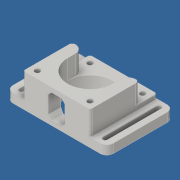
# Autodesk Inventor part: rotNema23Mount
Saved by Autodesk Inventor 2016 (Build 200138000, 138)
## iProperties
Created: 2015-10-04
Part Number: rotNema23Mount
Material: ABS-Kunststoff
Document SubType Name: Modeling
Designer: 4ndreas
Density: 1.06 g/cm^3
Appearance: Glatt - weiß
Mass: 62.6709 g
Surface Area: 197.225 cm^2
Volume: 59.1235 cm^3
Author: 4ndreas
Autodesk Inventor part; units mm, degrees
ref_plane "YZ Plane" through (0, 0, 0) normal (1, 0, 0) x (0, 1, 0)
sketch "Skizze1" plane through (0, 0, 0) normal (0, 0, 1) x (1, 0, 0)
  line L0 (-45, -30) -> (45, -30)
  line L1 (45, -30) -> (45, 30)
  line L2 (45, 30) -> (-45, 30)
  line L3 (-45, 30) -> (-45, -30)
  line L4 (-45, -30) -> (45, 30) construction
  line L5 (45, -30) -> (-45, 30) construction
  point P0 (0, 0)
  dimension "d0" = 60
  dimension "d1" = 90
  constraints: 12 end point, 2 midpoint, 2 parallel, 1 horizontal, 1 perpendicular
  measures "d0" distance between parallel lines of L0 L2
  measures "d1" distance between parallel lines of L3 L1
extrude "Extrusion1" add sketch "Skizze1" along normal blind 6
sketch "Skizze2" plane through (0, 0, 6) normal (0, 0, 1) x (1, 0, 0)
  line L0 (-30, -30) -> (30, -30)
  line L1 (30, -30) -> (30, 30)
  line L2 (30, 30) -> (-30, 30)
  line L3 (-30, 30) -> (-30, -30)
  line L4 (-30, -30) -> (30, 30) construction
  line L5 (30, -30) -> (-30, 30) construction
  line L6 (-45, -30) -> (45, -30) projected
  line L7 (45, -30) -> (45, 30) projected
  line L8 (45, 30) -> (-45, 30) projected
  line L9 (-45, 30) -> (-45, -30) projected
  line L10 (45, 30) -> (-45, 30) projected
  point P0 (0, 0)
  constraints: 12 end point, 2 midpoint, 2 parallel, 2 perpendicular, 1 collinear, 1 horizontal
sketch "Skizze3" plane through (0, 0, 0) normal (0, 0, -1) x (-1, 0, 0)
  line L0 (23.57, 23.57) -> (-23.57, 23.57) construction
  line L1 (-23.57, 23.57) -> (-23.57, -23.57) construction
  line L2 (-23.57, -23.57) -> (23.57, -23.57) construction
  line L3 (23.57, -23.57) -> (23.57, 23.57) construction
  line L4 (23.57, 23.57) -> (-23.57, -23.57) construction
  line L5 (-23.57, 23.57) -> (23.57, -23.57) construction
  point P0 (0, 0)
  dimension "d4" = 47.14
  constraints: 12 end point, 2 midpoint, 2 parallel, 2 perpendicular, 1 horizontal
  measures "d4" distance between parallel lines of L0 L2
extrude "Extrusion2" add sketch "Skizze2" along normal blind 14 contours L3 L2 L1 L0
hole "Bohrung1" at (-23.57, -23.57, 0) at (23.57, -23.57, 0) at (23.57, 23.57, 0) at (-23.57, 23.57, 0) direction (0, 0, 1) diameter 4.2 end through all
sketch "Skizze5" plane through (0, 0, 20) normal (0, 0, 1) x (1, 0, 0)
  circle A0 centre (0, 0) radius 20
  line L0 (-30, -30) -> (30, -30) projected
  line L1 (30, -30) -> (30, 30) projected
  line L2 (30, 30) -> (-30, 30) projected
  line L3 (-30, 30) -> (-30, -30) projected
  circle A1 centre (23.57, 23.57) radius 10
  circle A2 centre (-23.57, 23.57) radius 10
  line L4 (20, 0) -> (20, 14.229)
  line L5 (-20, 0) -> (-20, 14.229)
  line L6 (15.9113, 30) -> (-15.9113, 30)
  circle A3 centre (23.57, 23.57) radius 2.1 projected
  circle A4 centre (-23.57, 23.57) radius 2.1 projected
  dimension "d17" = 40
  dimension "d18" = 20
  constraints: 6 end point, 6 point on circle, 5 coincident, 3 centre point, 2 point on line, 2 tangent, 1 equal radius, 1 parallel, 1 vertical
  measures "d17" diameter of A0
  measures "d18" diameter of A1
extrude "Extrusion4" cut sketch "Skizze5" against normal blind 8 contours A0 | A0 L5 A2 L2 A1 L4 | A1 L2 L1 | A2 L3 L2 | A1 L1 L2 | A2 L2 L3 | A3 | A4
fillet "Rundung1" radius 7 2 edges at (20, 14.229, 16) (-20, 14.229, 16)
fillet "Rundung1" radius 3 2 edges at (-30, 15.9113, 16) (30, 15.9113, 16)
sketch "Skizze6" plane through (0, 0, 0) normal (0, 0, -1) x (-1, 0, 0)
  circle A0 centre (0, 0) radius 20
  dimension "d23" = 40
  constraints: 1 centre point, 1 coincident
  measures "d23" diameter of A0
extrude "Extrusion5" cut sketch "Skizze6" against normal through all
fillet "Rundung2" radius 6 4 edges at (45, -30, 3) (45, 30, 3) (-45, 30, 3) (-45, -30, 3)
sketch "Skizze7" plane through (0, 0, 20) normal (0, 0, 1) x (1, 0, 0)
  arc A0 (30, 11.0307) -> (26.2085, 13.9244) centre (27, 11.0307) ccw projected
  arc A1 (25.5876, 13.7757) -> (26.2085, 13.9244) centre (23.57, 23.57) ccw projected
  arc A2 (25.5876, 13.7757) -> (20, 6.9196) centre (27, 6.9196) ccw projected
  line L0 (20, 6.9196) -> (20, 0) projected
  arc A3 (-20, 0) -> (20, 0) centre (0, 0) ccw projected
  line L1 (-20, 0) -> (-20, 6.9196) projected
  arc A4 (-20, 6.9196) -> (-25.5876, 13.7757) centre (-27, 6.9196) ccw projected
  arc A5 (-26.2085, 13.9244) -> (-25.5876, 13.7757) centre (-23.57, 23.57) ccw projected
  arc A6 (-26.2085, 13.9244) -> (-30, 11.0307) centre (-27, 11.0307) ccw projected
  line L2 (-30, 11.0307) -> (-30, -30) projected
  line L3 (-30, -30) -> (30, -30) projected
  line L4 (30, -30) -> (30, 11.0307) projected
ref_plane "Arbeitsebene2" through (0, 0, 29.6) normal (0, 0, 1) x (1, 0, 0)
extrude "Extrusion6" add sketch "Skizze7" along normal up to surface (9.6 mm away)
sketch "Skizze8" plane through (-39, -30, 0) normal (0, -1, 0) x (1, 0, 0)
  line L0 (59, 0) -> (19, 0) projected
  line L1 (19, 12) -> (19, 29.6) projected
  line L2 (59, 29.6) -> (59, 12) projected
  line L3 (19, 12) -> (59, 12) projected
  line L4 (31.5, 4) -> (46.5, 4)
  line L5 (46.5, 4) -> (46.5, 25.6)
  line L6 (46.5, 25.6) -> (31.5, 25.6)
  line L7 (31.5, 25.6) -> (31.5, 4)
  line L8 (39, 29.6) -> (39, 12) construction
  line L9 (19, 29.6) -> (59, 29.6) projected
  point P0 (39, 0)
  dimension "d32" = 4
  dimension "d33" = 15
  constraints: 10 end point, 2 parallel, 1 horizontal, 1 midpoint, 1 perpendicular, 1 other
  measures "d32" distance between parallel lines of L0 L4
  measures "d33" distance between parallel lines of L7 L5
extrude "Extrusion7" cut sketch "Skizze8" against normal blind 30 contours L7 L6 L5 L3 | L3 L5 L4 L7
chamfer "Fase1" distance 3 angle 45 4 edges at (-7.5, -24.2702, 4) (7.5, -24.2702, 4) (7.5, -24.2702, 25.6) (-7.5, -24.2702, 25.6)
sketch "Skizze10" plane through (0, 0, 6) normal (0, 0, 1) x (1, 0, 0)
  arc A0 (45, 24) -> (39, 30) centre (39, 24) ccw projected
  line L0 (39, 30) -> (30, 30) projected
  line L1 (30, 30) -> (30, -30) projected
  line L2 (30, -30) -> (39, -30) projected
  arc A1 (39, -30) -> (45, -24) centre (39, -24) ccw projected
  line L3 (45, -24) -> (45, 24) projected
  arc A2 (-45, -24) -> (-39, -30) centre (-39, -24) ccw projected
  line L4 (-39, -30) -> (-30, -30) projected
  line L5 (-30, -30) -> (-30, 30) projected
  line L6 (-30, 30) -> (-39, 30) projected
  arc A3 (-39, 30) -> (-45, 24) centre (-39, 24) ccw projected
  line L7 (-45, 24) -> (-45, -24) projected
  line L8 (37.5, 26) -> (37.5, -26) construction
  line L9 (39.5, 24) -> (39.5, -24)
  line L10 (35.5, -24) -> (35.5, 24)
  arc A4 (39.5, 24) -> (35.5, 24) centre (37.5, 24) ccw
  arc A5 (35.5, -24) -> (39.5, -24) centre (37.5, -24) ccw
  line L11 (45, 0) -> (-45, 0) construction
  circle A6 centre (37.5, 0) radius 7.5 construction
  point P0 (0, 0)
  dimension "d42" = 4
  dimension "d44" = 48
  constraints: 10 end point, 6 point on circle, 6 tangent, 3 centre point, 3 midpoint, 3 point on line, 1 coincident, 1 parallel, 1 vertical
  measures "d42" distance between parallel lines of L9 L10
  measures "d44" distance of A4.centre A5.centre
extrude "Extrusion9" cut sketch "Skizze10" against normal through all contours L9 A5 L10 A4
ref_plane "Arbeitsebene3" through (0, -24, 0) normal (1, 0, 0) x (0, 0, -1)
mirror "Spiegeln1" about plane through (0, -24, 0) normal (1, 0, 0) of "Extrusion9"
hole "Bohrung2" at (-23.57, -23.57, 0) at (23.57, -23.57, 0) at (23.57, 23.57, 0) at (-23.57, 23.57, 0) direction (0, 0, 1) diameter 4.5 end through all
sketch "Skizze11" plane through (0, 0, 0) normal (0, 0, -1) x (-1, 0, 0)
  circle A0 centre (-23.57, 23.57) radius 2.25 projected
  circle A1 centre (23.57, -23.57) radius 2.25 projected
  circle A2 centre (-23.57, -23.57) radius 2.25 projected
  circle A3 centre (23.57, 23.57) radius 2.25 projected
  arc A4 (35.5, -24) -> (39.5, -24) centre (37.5, -24) ccw projected
  line L0 (35.5, -24) -> (35.5, 24) projected
  arc A5 (39.5, 24) -> (35.5, 24) centre (37.5, 24) ccw projected
  line L1 (39.5, 24) -> (39.5, -24) projected
  arc A6 (-35.5, 24) -> (-39.5, 24) centre (-37.5, 24) ccw projected
  line L2 (-35.5, 24) -> (-35.5, -24) projected
  arc A7 (-39.5, -24) -> (-35.5, -24) centre (-37.5, -24) ccw projected
  line L3 (-39.5, -24) -> (-39.5, 24) projected
  arc A8 (39, -30) -> (45, -24) centre (39, -24) ccw projected
  line L4 (45, 24) -> (45, -24) projected
  arc A9 (45, 24) -> (39, 30) centre (39, 24) ccw projected
  line L5 (-39, 30) -> (39, 30) projected
  arc A10 (-39, 30) -> (-45, 24) centre (-39, 24) ccw projected
  line L6 (-45, -24) -> (-45, 24) projected
  arc A11 (-45, -24) -> (-39, -30) centre (-39, -24) ccw projected
  line L7 (39, -30) -> (-39, -30) projected
  circle A12 centre (0, 0) radius 20 projected
  line L8 (27.6115, 23.57) -> (25.5907, 20.07)
  line L9 (25.5907, 20.07) -> (21.5493, 20.07)
  line L10 (21.5493, 20.07) -> (19.5285, 23.57)
  line L11 (19.5285, 23.57) -> (21.5493, 27.07)
  line L12 (21.5493, 27.07) -> (25.5907, 27.07)
  line L13 (25.5907, 27.07) -> (27.6115, 23.57)
  line L14 (-19.5285, 23.57) -> (-21.5493, 20.07)
  line L15 (-21.5493, 20.07) -> (-25.5907, 20.07)
  line L16 (-25.5907, 20.07) -> (-27.6115, 23.57)
  line L17 (-27.6115, 23.57) -> (-25.5907, 27.07)
  line L18 (-25.5907, 27.07) -> (-21.5493, 27.07)
  line L19 (-21.5493, 27.07) -> (-19.5285, 23.57)
  line L20 (-19.5285, -23.57) -> (-21.5493, -27.07)
  line L21 (-21.5493, -27.07) -> (-25.5907, -27.07)
  line L22 (-25.5907, -27.07) -> (-27.6115, -23.57)
  line L23 (-27.6115, -23.57) -> (-25.5907, -20.07)
  line L24 (-25.5907, -20.07) -> (-21.5493, -20.07)
  line L25 (-21.5493, -20.07) -> (-19.5285, -23.57)
  line L26 (19.5285, -23.57) -> (21.5493, -20.07)
  line L27 (21.5493, -20.07) -> (25.5907, -20.07)
  line L28 (25.5907, -20.07) -> (27.6115, -23.57)
  line L29 (27.6115, -23.57) -> (25.5907, -27.07)
  line L30 (25.5907, -27.07) -> (21.5493, -27.07)
  line L31 (21.5493, -27.07) -> (19.5285, -23.57)
  line L32 (-39, 30) -> (39, 30) projected
  line L33 (39, -30) -> (-39, -30) projected
  dimension "d54" = 7
  constraints: 48 end point, 4 coincident, 4 parallel, 3 equal length, 52 other
  measures "d54" distance between parallel lines of L12 L9
extrude "Extrusion10" cut sketch "Skizze11" against normal blind 4 contours A0 | A1 | A2 | A3 | L8 L9 L10 L11 L12 L13 | L14 L15 L16 L17 L18 L19 | L20 L21 L22 L23 L24 L25 | L26 L27 L28 L29 L30 L31
sketch "Skizze12" plane through (0, 0, 4) normal (0, 0, -1) x (-1, 0, 0)
  circle A0 centre (23.57, 23.57) radius 2.25 projected
  circle A1 centre (23.57, -23.57) radius 2.25 projected
  circle A2 centre (-23.57, -23.57) radius 2.25 projected
  circle A3 centre (-23.57, 23.57) radius 2.25 projected
  point P0 (0, 0)
extrude "Extrusion11" add sketch "Skizze12" against normal blind 0.2
fillet "Rundung3" radius 2 4 edges at (30, -30, 17.8) (-30, -30, 17.8) (30, 30, 9) (-30, 30, 9)
sketch "Skizze13" plane through (0, 0, 6) normal (0, 0, 1) x (1, 0, 0)
  arc A0 (-39.5, -24) -> (-35.5, -24) centre (-37.5, -24) ccw projected
  line L0 (-39.5, -24) -> (-39.5, 24) projected
  arc A1 (-35.5, 24) -> (-39.5, 24) centre (-37.5, 24) ccw projected
  line L1 (-35.5, 24) -> (-35.5, -24) projected
  arc A2 (-45, -24) -> (-39, -30) centre (-39, -24) ccw projected
  line L2 (-39, -30) -> (-28, -30) projected
  arc A3 (-30, -28) -> (-28, -30) centre (-28, -28) ccw projected
  line L3 (-30, -28) -> (-30, 28) projected
  arc A4 (-28, 30) -> (-30, 28) centre (-28, 28) ccw projected
  line L4 (-28, 30) -> (-39, 30) projected
  arc A5 (-39, 30) -> (-45, 24) centre (-39, 24) ccw projected
  line L5 (-45, 24) -> (-45, -24) projected
  arc A6 (39.5, 24) -> (35.5, 24) centre (37.5, 24) ccw projected
  line L6 (39.5, 24) -> (39.5, -24) projected
  arc A7 (35.5, -24) -> (39.5, -24) centre (37.5, -24) ccw projected
  line L7 (35.5, -24) -> (35.5, 24) projected
  arc A8 (45, 24) -> (39, 30) centre (39, 24) ccw projected
  line L8 (39, 30) -> (28, 30) projected
  arc A9 (30, 28) -> (28, 30) centre (28, 28) ccw projected
  line L9 (30, 28) -> (30, -28) projected
  arc A10 (28, -30) -> (30, -28) centre (28, -28) ccw projected
  line L10 (28, -30) -> (39, -30) projected
  arc A11 (39, -30) -> (45, -24) centre (39, -24) ccw projected
  line L11 (45, -24) -> (45, 24) projected
  point P0 (0, 0)
extrude "Extrusion12" add sketch "Skizze13" along normal blind 2
